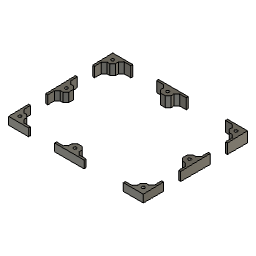
support (Autodesk Fusion 360 design; units mm, degrees)
Autodesk Fusion 360 part; units mm, degrees
note: some values were not read from the file. Chosen so that the rebuilt part matches the saved one: which bodies a step acts on.
sketch "Sketch1" plane through (0, 0, 0) normal (0, 0, 1) x (1, 0, 0)
  line L0 (0, 0) -> (287.292, 0)
  line L1 (287.292, 0) -> (287.292, -2.5)
  line L2 (287.292, -2.5) -> (0, -2.5)
  line L3 (0, -2.5) -> (0, 0)
  line L4 (0, -2.5) -> (2.5, -2.5)
  line L5 (2.5, -2.5) -> (2.5, -220.5)
  line L6 (2.5, -220.5) -> (0, -220.5)
  line L7 (0, -220.5) -> (0, -2.5)
  line L8 (287.292, -2.5) -> (284.792, -2.5)
  line L9 (284.792, -2.5) -> (284.792, -220.5)
  line L10 (284.792, -220.5) -> (287.292, -220.5)
  line L11 (287.292, -220.5) -> (287.292, -2.5)
  line L12 (0, -220.5) -> (287.292, -220.5)
  line L13 (287.292, -220.5) -> (287.292, -223)
  line L14 (287.292, -223) -> (0, -223)
  line L15 (0, -223) -> (0, -220.5)
  line L16 (2.5, -2.5) -> (24.5, -2.5)
  line L17 (24.5, -2.5) -> (24.5, -24.5)
  line L18 (24.5, -24.5) -> (2.5, -24.5)
  line L19 (2.5, -24.5) -> (2.5, -2.5)
  line L20 (24.5, -2.5) -> (44.5, -2.5)
  line L21 (44.5, -2.5) -> (44.5, -6.5)
  line L22 (44.5, -6.5) -> (24.5, -6.5)
  line L23 (24.5, -6.5) -> (24.5, -2.5)
  line L24 (2.5, -24.5) -> (6.5, -24.5)
  line L25 (6.5, -24.5) -> (6.5, -44.5)
  line L26 (6.5, -44.5) -> (2.5, -44.5)
  line L27 (2.5, -44.5) -> (2.5, -24.5)
  circle A0 centre (14.5, -14.5) radius 3
  line L28 (2.5, -220.5) -> (24.5, -220.5)
  line L29 (24.5, -220.5) -> (24.5, -198.5)
  line L30 (24.5, -198.5) -> (2.5, -198.5)
  line L31 (2.5, -198.5) -> (2.5, -220.5)
  line L32 (2.5, -198.5) -> (6.5, -198.5)
  line L33 (6.5, -198.5) -> (6.5, -178.5)
  line L34 (6.5, -178.5) -> (2.5, -178.5)
  line L35 (2.5, -178.5) -> (2.5, -198.5)
  line L36 (24.5, -220.5) -> (44.5, -220.5)
  line L37 (44.5, -220.5) -> (44.5, -216.5)
  line L38 (44.5, -216.5) -> (24.5, -216.5)
  line L39 (24.5, -216.5) -> (24.5, -220.5)
  circle A1 centre (14.5, -208.5) radius 3
  circle A2 centre (14.5, -111.5) radius 3
  line L40 (2.5, -100.5) -> (24.5, -100.5)
  line L41 (24.5, -100.5) -> (24.5, -122.5)
  line L42 (24.5, -122.5) -> (2.5, -122.5)
  line L43 (2.5, -122.5) -> (2.5, -100.5)
  line L44 (2.5, -100.5) -> (6.5, -100.5)
  line L45 (6.5, -100.5) -> (6.5, -80.5)
  line L46 (6.5, -80.5) -> (2.5, -80.5)
  line L47 (2.5, -80.5) -> (2.5, -100.5)
  line L48 (2.5, -122.5) -> (6.5, -122.5)
  line L49 (6.5, -122.5) -> (6.5, -142.5)
  line L50 (6.5, -142.5) -> (2.5, -142.5)
  line L51 (2.5, -142.5) -> (2.5, -122.5)
  line L52 (118.7731, -243) -> (140.7731, -243)
  line L53 (140.7731, -243) -> (140.7731, -265)
  line L54 (140.7731, -265) -> (118.7731, -265)
  line L55 (118.7731, -265) -> (118.7731, -243)
  line L56 (140.7731, -243) -> (160.7731, -243)
  line L57 (160.7731, -243) -> (160.7731, -247)
  line L58 (160.7731, -247) -> (140.7731, -247)
  line L59 (140.7731, -247) -> (140.7731, -243)
  line L60 (118.7731, -243) -> (98.7731, -243)
  line L61 (98.7731, -243) -> (98.7731, -247)
  line L62 (98.7731, -247) -> (118.7731, -247)
  line L63 (118.7731, -247) -> (118.7731, -243)
  circle A3 centre (129.7731, -255) radius 3
  line L64 (118.7731, -439) -> (140.7731, -439)
  line L65 (140.7731, -439) -> (140.7731, -461)
  line L66 (140.7731, -461) -> (118.7731, -461)
  line L67 (118.7731, -461) -> (118.7731, -439)
  line L68 (118.7731, -461) -> (98.7731, -461)
  line L69 (98.7731, -461) -> (98.7731, -457)
  line L70 (98.7731, -457) -> (118.7731, -457)
  line L71 (118.7731, -457) -> (118.7731, -461)
  line L72 (140.7731, -461) -> (160.7731, -461)
  line L73 (160.7731, -461) -> (160.7731, -457)
  line L74 (160.7731, -457) -> (140.7731, -457)
  line L75 (140.7731, -457) -> (140.7731, -461)
  circle A4 centre (129.7731, -449) radius 3
  dimension "d1" = 287.292
  dimension "d2" = 2.5
  dimension "d3" = 2.5
  dimension "d4" = 218
  dimension "d5" = 2.5
  dimension "d6" = 218
  dimension "d7" = 2.5
  dimension "d8" = 22
  dimension "d9" = 22
  dimension "d10" = 20
  dimension "d11" = 4
  dimension "d12" = 4
  dimension "d13" = 20
  dimension "d14" = 6
  dimension "d15" = 10
  dimension "d16" = 10
  dimension "d17" = 22
  dimension "d18" = 22
  dimension "d19" = 4
  dimension "d20" = 20
  dimension "d21" = 20
  dimension "d22" = 4
  dimension "d23" = 6
  dimension "d24" = 10
  dimension "d25" = 10
  dimension "d26" = 97
  dimension "d27" = 6
  dimension "d28" = 22
  dimension "d29" = 22
  dimension "d30" = 10
  dimension "d31" = 11
  dimension "d32" = 4
  dimension "d33" = 20
  dimension "d34" = 4
  dimension "d35" = 20
  dimension "d58" = 22
  dimension "d59" = 22
  dimension "d60" = 20
  dimension "d61" = 4
  dimension "d62" = 20
  dimension "d63" = 4
  dimension "d64" = 6
  dimension "d65" = 11
  dimension "d66" = 10
  dimension "d67" = 22
  dimension "d68" = 22
  dimension "d69" = 20
  dimension "d70" = 4
  dimension "d71" = 20
  dimension "d72" = 4
  dimension "d73" = 6
  dimension "d74" = 10
  dimension "d75" = 11
  dimension "d76" = 218
  constraint horizontal L0
  constraint vertical L1
  constraint horizontal L2
  constraint vertical L3
  constraint coincident L0.start L3.end
  constraint horizontal L4
  constraint vertical L5
  constraint horizontal L6
  constraint vertical L7
  constraint horizontal L8
  constraint vertical L9
  constraint horizontal L10
  constraint vertical L11
  constraint horizontal L12
  constraint vertical L13
  constraint horizontal L14
  constraint vertical L15
  constraint horizontal L16
  constraint vertical L17
  constraint horizontal L18
  constraint vertical L19
  constraint horizontal L20
  constraint vertical L21
  constraint horizontal L22
  constraint vertical L23
  constraint horizontal L24
  constraint vertical L25
  constraint horizontal L26
  constraint vertical L27
  constraint horizontal L28
  constraint vertical L29
  constraint horizontal L30
  constraint vertical L31
  constraint horizontal L32
  constraint vertical L33
  constraint horizontal L34
  constraint vertical L35
  constraint horizontal L36
  constraint vertical L37
  constraint horizontal L38
  constraint vertical L39
  constraint horizontal L40
  constraint vertical L41
  constraint horizontal L42
  constraint vertical L43
  constraint coincident L5 L40.start
  constraint horizontal L44
  constraint vertical L45
  constraint horizontal L46
  constraint vertical L47
  constraint horizontal L48
  constraint vertical L49
  constraint horizontal L50
  constraint vertical L51
  constraint horizontal L52
  constraint vertical L53
  constraint horizontal L54
  constraint vertical L55
  constraint horizontal L56
  constraint vertical L57
  constraint horizontal L58
  constraint vertical L59
  constraint horizontal L60
  constraint vertical L61
  constraint horizontal L62
  constraint vertical L63
  constraint horizontal L64
  constraint vertical L65
  constraint horizontal L66
  constraint vertical L67
  constraint horizontal L68
  constraint vertical L69
  constraint horizontal L70
  constraint vertical L71
  constraint horizontal L72
  constraint vertical L73
  constraint horizontal L74
  constraint vertical L75
  measures "d1" distance of L0.start L0.end
  measures "d2" distance of L0.start L2.end
  measures "d3" distance of L2.end L4.end
  measures "d4" distance of L2.end L6.end
  measures "d5" distance of L1.end L8.end
  measures "d6" distance of L1.end L10.end
  measures "d7" distance of L6.end L14.end
  measures "d8" distance of L4.end L16.end
  measures "d9" distance of L4.end L18.end
  measures "d10" distance of L16.end L20.end
  measures "d11" distance of L16.end L22.end
  measures "d12" distance of L18.end L24.end
  measures "d13" distance of L18.end L26.end
  measures "d14" diameter of A0
  measures "d15" distance of L17 A0.centre
  measures "d16" distance of L18 A0.centre
  measures "d17" distance of L5.end L28.end
  measures "d18" distance of L5.end L30.end
  measures "d19" distance of L30.end L32.end
  measures "d20" distance of L30.end L34.end
  measures "d21" distance of L28.end L36.end
  measures "d22" distance of L28.end L38.end
  measures "d23" diameter of A1
  measures "d24" distance of L30 A1.centre
  measures "d25" distance of L29 A1.centre
  measures "d26" distance of A0.centre A2.centre
  measures "d27" diameter of A2
  measures "d28" distance of L40.start L40.end
  measures "d29" distance of L40.start L42.end
  measures "d30" distance of A2.centre L41
  measures "d31" distance of A2.centre L40
  measures "d32" distance of L40.start L44.end
  measures "d33" distance of L40.start L46.end
  measures "d34" distance of L42.end L48.end
  measures "d35" distance of L42.end L50.end
  measures "d58" distance of L52.start L52.end
  measures "d59" distance of L52.start L54.end
  measures "d60" distance of L52.end L56.end
  measures "d61" distance of L52.end L58.end
  measures "d62" distance of L52.start L60.end
  measures "d63" distance of L52.start L62.end
  measures "d64" diameter of A3
  measures "d65" distance of L53 A3.centre
  measures "d66" distance of L54 A3.centre
  measures "d67" distance of L64.start L64.end
  measures "d68" distance of L64.start L66.end
  measures "d69" distance of L66.end L68.end
  measures "d70" distance of L66.end L70.end
  measures "d71" distance of L65.end L72.end
  measures "d72" distance of L65.end L74.end
  measures "d73" diameter of A4
  measures "d74" distance of L64 A4.centre
  measures "d75" distance of L67 A4.centre
  measures "d76" distance of L52 L66
extrude "Extrude1" add sketch "Sketch1" along normal blind 22 contours L2 L5 L16 L17 L18 L19 L23 L24 | L2 L17 L20 L21 L22 L23 | L5 L18 L24 L25 L26 L27 makes body 1
extrude "Extrude2" add sketch "Sketch1" along normal blind 18 separate body contours L5 L12 L28 L29 L30 L31 L32 L39 | L5 L30 L32 L33 L34 L35 | L12 L29 L36 L37 L38 L39 makes body 2
extrude "Extrude3" add sketch "Sketch1" along normal blind 22 separate body contours L5 L40 L44 L45 L46 L47 | L5 L40 L41 L42 L43 L44 L48 | L5 L42 L48 L49 L50 L51 makes body 3
sketch "Sketch2" plane through (2.5, 0, 0) normal (-1, 0, 0) x (0, -1, 0)
  line L0 (2.5, 0) -> (44.5, 0)
  line L1 (44.5, 0) -> (44.5, 22)
  line L2 (44.5, 22) -> (2.5, 22)
  line L3 (2.5, 22) -> (2.5, 0)
  line L4 (2.5, 0) -> (220.5, 0)
  line L5 (220.5, 0) -> (220.5, 16)
  line L6 (220.5, 16) -> (2.5, 22)
  dimension "d42" = 218
  dimension "d43" = 16
  constraint coincident L0.start L3.end
  constraint perpendicular L3 L4
  constraint perpendicular L4 L5
  constraint coincident L2.end L3.start
  measures "d42" distance of L0.start L4.end
  measures "d43" distance of L4.end L5.end
extrude "Extrude4" cut sketch "Sketch2" against normal through all contours L1 L2 L6 bodies 1
sketch "Sketch3" plane through (2.5, 0, 0) normal (-1, 0, 0) x (0, -1, 0)
  line L0 (178.5, 0) -> (220.5, 0)
  line L1 (220.5, 0) -> (220.5, 18)
  line L2 (220.5, 18) -> (178.5, 18)
  line L3 (178.5, 18) -> (178.5, 0)
  line L4 (220.5, 0) -> (2.5, 0)
  line L5 (2.5, 0) -> (2.5, 22)
  line L6 (220.5, 0) -> (220.5, 16)
  line L7 (220.5, 16) -> (2.5, 22)
  dimension "d45" = 218
  dimension "d46" = 22
  dimension "d47" = 16
  constraint coincident L0.end L1.start
  constraint perpendicular L1 L4
  constraint perpendicular L4 L5
  constraint perpendicular L4 L6
  measures "d45" distance of L0.end L4.end
  measures "d46" distance of L4.end L5.end
  measures "d47" distance of L0.end L6.end
extrude "Extrude5" cut sketch "Sketch3" against normal through all contours L1 L2 L3 L7 bodies 2
sketch "Sketch4" plane through (2.5, 0, 0) normal (-1, 0, 0) x (0, -1, 0)
  line L0 (80.5, 0) -> (142.5, 0)
  line L1 (142.5, 0) -> (142.5, 22)
  line L2 (142.5, 22) -> (80.5, 22)
  line L3 (80.5, 22) -> (80.5, 0)
  line L4 (0, 0) -> (2.5, 0)
  line L5 (2.5, 0) -> (220.5, 0)
  line L6 (2.5, 0) -> (2.5, 22)
  line L7 (220.5, 0) -> (220.5, 16)
  line L8 (220.5, 16) -> (2.5, 22)
  dimension "d49" = 2.5
  dimension "d50" = 218
  dimension "d51" = 22
  dimension "d52" = 16
  constraint coincident L4.start origin
  constraint horizontal L4
  constraint parallel L4 L5
  constraint perpendicular L5 L6
  constraint perpendicular L5 L7
  measures "d49" distance of L4.start L4.end
  measures "d50" distance of L4.end L5.end
  measures "d51" distance of L4.end L6.end
  measures "d52" distance of L5.end L7.end
extrude "Extrude6" cut sketch "Sketch4" against normal through all contours L1 L2 L3 L8 bodies 3
mirror "Mirror1" about plane through (0, 0, 0) normal (1, 0, 0) of bodies 1 3 2 makes body 4 at (-30.5, -2.5, 7.3333) makes body 5 at (-2.5, -192.5, 11.052) makes body 6 at (-2.5, -101.1667, 12.6667)
move_body "Move1" bodies 4 6 5 to x (1, 0, 0) y (0, 1, 0) z (0, 0, 1) at (287.2, 0, 0)
extrude "Extrude7" add sketch "Sketch1" along normal blind 22 separate body contours L52 L53 L54 L55 L59 L63 | L55 L60 L61 L62 L63 | L53 L56 L57 L58 L59 | L64 L65 L66 L67 L71 L75 | L67 L68 L69 L70 L71 | L65 L72 L73 L74 L75 makes body 7 at (119.4397, -243, 7.3333) makes body 8 at (140.1064, -461, 14.6667)
sketch "Sketch5" plane through (98.7731, 0, 0) normal (-1, 0, 0) x (0, -1, 0)
  line L0 (243, 0) -> (247, 0)
  line L1 (247, 0) -> (247, 22)
  line L2 (247, 22) -> (243, 22)
  line L3 (243, 22) -> (243, 0)
  line L4 (243, 0) -> (461, 0)
  line L5 (461, 0) -> (461, 16)
  line L6 (461, 16) -> (243, 22)
  dimension "d80" = 218
  dimension "d81" = 16
  constraint coincident L0.start L3.end
  constraint perpendicular L3 L4
  constraint perpendicular L4 L5
  constraint coincident L2.end L3.start
  measures "d80" distance of L0.start L4.end
  measures "d81" distance of L4.end L5.end
sketch "Sketch6" plane through (118.7731, 0, 0) normal (-1, 0, 0) x (0, -1, 0)
  line L0 (247, 0) -> (265, 0)
  line L1 (265, 0) -> (265, 22)
  line L2 (265, 22) -> (247, 22)
  line L3 (247, 22) -> (247, 0)
  line L4 (247, 0) -> (243, 0)
  line L5 (243, 0) -> (243, 22)
  line L6 (243, 0) -> (461, 0)
  line L7 (461, 0) -> (461, 16)
  line L8 (461, 16) -> (243, 22)
  dimension "d82" = 4
  dimension "d83" = 22
  dimension "d84" = 218
  dimension "d85" = 16
  constraint coincident L0.start L3.end
  constraint perpendicular L3 L4
  constraint perpendicular L4 L5
  constraint perpendicular L5 L6
  constraint perpendicular L6 L7
  measures "d82" distance of L0.start L4.end
  measures "d83" distance of L4.end L5.end
  measures "d84" distance of L4.end L6.end
  measures "d85" distance of L6.end L7.end
extrude "Extrude8" cut sketch "Sketch5" against normal through all contours L1 L2 L6 bodies 7
extrude "Extrude9" cut sketch "Sketch6" against normal through all contours L1 L2 L3 L8 bodies 7
sketch "Sketch7" plane through (98.7731, 0, 0) normal (-1, 0, 0) x (0, -1, 0)
  line L0 (457, 0) -> (461, 0)
  line L1 (461, 0) -> (461, 22)
  line L2 (461, 22) -> (457, 22)
  line L3 (457, 22) -> (457, 0)
  line L4 (461, 0) -> (243, 0)
  line L5 (243, 0) -> (243, 22)
  line L6 (461, 0) -> (461, 16)
  line L7 (461, 16) -> (243, 22)
  dimension "d88" = 218
  dimension "d89" = 22
  dimension "d90" = 16
  constraint coincident L0.end L1.start
  constraint perpendicular L1 L4
  constraint perpendicular L4 L5
  constraint perpendicular L4 L6
  measures "d88" distance of L0.end L4.end
  measures "d89" distance of L4.end L5.end
  measures "d90" distance of L0.end L6.end
sketch "Sketch8" plane through (118.7731, 0, 0) normal (-1, 0, 0) x (0, -1, 0)
  line L0 (439, 0) -> (457, 0)
  line L1 (457, 0) -> (457, 22)
  line L2 (457, 22) -> (439, 22)
  line L3 (439, 22) -> (439, 0)
  line L4 (457, 0) -> (461, 0)
  line L5 (461, 0) -> (461, 16)
  line L6 (461, 0) -> (243, 0)
  line L7 (243, 0) -> (243, 22)
  line L8 (243, 22) -> (461, 16)
  dimension "d91" = 4
  dimension "d92" = 16
  dimension "d93" = 218
  dimension "d94" = 22
  constraint coincident L0.end L1.start
  constraint perpendicular L1 L4
  constraint perpendicular L4 L5
  constraint perpendicular L5 L6
  constraint perpendicular L6 L7
  measures "d91" distance of L0.end L4.end
  measures "d92" distance of L4.end L5.end
  measures "d93" distance of L4.end L6.end
  measures "d94" distance of L6.end L7.end
extrude "Extrude10" cut sketch "Sketch7" against normal through all contours L1 L2 L3 L7 bodies 8
extrude "Extrude11" cut sketch "Sketch8" against normal through all contours L1 L2 L3 L8 bodies 8
move_body "Move2" bodies 7 8 to x (1, 0, 0) y (0, 1, 0) z (0, 0, 1) at (0, 240.4, 0)
chamfer "Chamfer2" distance 6 angle 45 28 edges at (280.7, -122.5, 9.3486) (280.7, -100.5, 9.6514) (262.7, -100.5, 9.6514) (262.7, -122.5, 9.3486) (140.7731, -6.6, 10.945) (140.7731, -24.6, 10.6972) (118.7731, -24.6, 10.6972) (118.7731, -6.6, 10.945) (6.5, -198.5, 8.3028) (24.5, -198.5, 8.3028) (24.5, -216.5, 8.055) (262.7, -216.5, 8.055) (262.7, -198.5, 8.3028) (280.7, -198.5, 8.3028) (24.5, -6.5, 10.945) (24.5, -24.5, 10.6972) (6.5, -24.5, 10.6972) (280.7, -24.5, 10.6972) (262.7, -24.5, 10.6972) (262.7, -6.5, 10.945) (118.7731, -216.6, 8.055) (118.7731, -198.6, 8.3028) (140.7731, -198.6, 8.3028) (140.7731, -216.6, 8.055) (6.5, -100.5, 9.6514) (24.5, -100.5, 9.6514) (24.5, -122.5, 9.3486) (6.5, -122.5, 9.3486) on bodies 1 2 3 4 5 6 7 8
